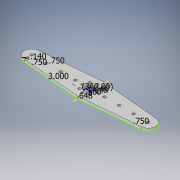
# Autodesk Inventor part: servoAttachment
Saved by Autodesk Inventor 2018 (Build 220112000, 112)
## iProperties
Created: 2017-10-15
Part Number: servoAttachment
Material: Generic
Document SubType Name: Modeling
Designer: snipe
Density: 1 g/cm^3
Appearance: Default
Author: snipe
Autodesk Inventor part; units mm, degrees
ref_plane "YZ Plane" through (0, 0, 0) normal (1, 0, 0) x (0, 1, 0)
ref_plane "XZ Plane" through (0, 0, 0) normal (0, 1, 0) x (-1, 0, 0)
ref_plane "XY Plane" through (0, 0, 0) normal (0, 0, 1) x (1, 0, 0)
sketch "Sketch1" plane through (0, 0, 0) normal (0, 1, 0) x (-1, 0, 0)
  line L0 (0, -23.0251) -> (0, 23.0251) projected
  line L1 (0, -23.0251) -> (0, 23.0251) projected
  circle A0 centre (0, 0) radius 6.35
  circle A1 centre (0, -9.779) radius 1.778
  circle A2 centre (6.9148, -6.9148) radius 1.778
  circle A3 centre (9.779, 0) radius 1.778
  circle A4 centre (6.9148, 6.9148) radius 1.778
  circle A5 centre (0, 9.779) radius 1.778
  circle A6 centre (-6.9148, 6.9148) radius 1.778
  circle A7 centre (-9.779, 0) radius 1.778
  circle A8 centre (-6.9148, -6.9148) radius 1.778
  line L2 (0, 0) -> (-76.2, 0)
  line L3 (0, 0) -> (76.2, 0)
  circle A9 centre (76.2, 0) radius 1.778
  circle A10 centre (57.15, 0) radius 1.778
  circle A11 centre (38.1, 0) radius 1.778
  circle A12 centre (19.05, 0) radius 1.778
  circle A13 centre (-76.2, 0) radius 1.778
  circle A14 centre (-57.15, 0) radius 1.778
  circle A15 centre (-38.1, 0) radius 1.778
  circle A16 centre (-19.05, 0) radius 1.778
  arc A17 (76.2, -9.525) -> (76.2, 9.525) centre (76.2, 0) ccw
  arc A18 (76.2, -9.525) -> (76.2, 9.525) centre (76.2, 0) ccw
  line L4 (66.675, 0) -> (76.2, 0) construction
  line L5 (0, 0) -> (11.557, 0) construction
  line L6 (76.2, -9.525) -> (0, -16.4465)
  line L7 (76.2, 9.525) -> (0, 16.4465)
  line L8 (0, 0) -> (-76.2, 0)
  circle A19 centre (-76.2, 0) radius 1.778
  circle A20 centre (-57.15, 0) radius 1.778
  circle A21 centre (-38.1, 0) radius 1.778
  circle A22 centre (-19.05, 0) radius 1.778
  arc A23 (-76.2, 9.525) -> (-76.2, -9.525) centre (-76.2, 0) ccw
  arc A24 (-76.2, 9.525) -> (-76.2, -9.525) centre (-76.2, 0) ccw
  line L9 (-66.675, 0) -> (-76.2, 0) construction
  line L10 (-76.2, -9.525) -> (0, -16.4465)
  line L11 (-76.2, 9.525) -> (0, 16.4465)
  line L12 (0, 16.4465) -> (0, -16.4465)
  circle A25 centre (0, 9.779) radius 1.778
  circle A26 centre (0, -9.779) radius 1.778
  circle A27 centre (0, 0) radius 6.35
  dimension "d0" = 12.7
  dimension "d2" = 3.556
  dimension "d5" = 360
  dimension "d8" = 76.2
  dimension "d10" = 16.4465
  dimension "d11" = 16.4465
  dimension "d12" = 3.556
  dimension "d15" = 19.05
  dimension "d23" = 19.05
  dimension "d29" = 19.05
  constraints: 27 centre point, 22 end point, 12 coincident, 11 symmetric about line, 8 point on circle, 4 horizontal, 3 point on line, 1 collinear, 1 horizontal alignment, 1 perpendicular, 37 other
  measures "d0" diameter of A0
  measures "d2" diameter of A1
  measures "d8" distance of L2.start L3.end
  measures "d10" distance of L2.start L6.end
  measures "d11" distance of L2.start L7.end
  measures "d12" diameter of A9
  measures "d15" distance of A9.centre A10.centre
  measures "d23" distance of A13.centre A14.centre
  measures "d29" diameter of A17
extrude "Extrusion2" add sketch "Sketch1" along normal blind 3.175
extrude "Extrusion3" cut sketch "Sketch1" along normal through all contours A1 L0 | L0 A1 | A0 L2 L0 | L0 L3 A0 | L2 A0 L0 | L0 A0 L3 | A5 L0 | L0 A5
body "Solid2"
